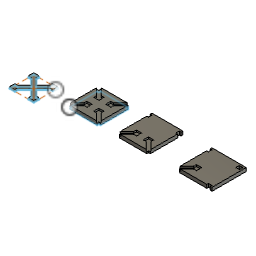
Maze_Alle_Module (Autodesk Fusion 360 design; units mm, degrees)
Autodesk Fusion 360 part; units mm, degrees
(part 1 of 2)
sketch "Skizze1" plane through (0, 0, 0) normal (0, 1, 0) x (1, 0, 0)
  line L0 (5, 0) -> (85, 0)
  line L1 (85, 0) -> (85, 5)
  line L2 (85, 5) -> (90, 5)
  line L3 (90, 5) -> (90, 85)
  line L4 (90, 85) -> (85, 85)
  line L5 (85, 85) -> (85, 90)
  line L6 (85, 90) -> (5, 90)
  line L7 (5, 90) -> (5, 85)
  line L8 (5, 85) -> (0, 85)
  line L9 (0, 85) -> (0, 5)
  line L10 (0, 5) -> (5, 5)
  line L11 (5, 5) -> (5, 0)
  line L12 (-35, 35) -> (35, 35) construction
  line L13 (35, 35) -> (35, -35) construction
  line L14 (35, -35) -> (-35, -35) construction
  line L15 (-35, -35) -> (-35, 35) construction
  line L16 (-35, 35) -> (35, -35) construction
  line L17 (35, 35) -> (-35, -35) construction
  line L18 (0, 0) -> (-3.5355, 3.5355) construction
  line L19 (-3.5355, 3.5355) -> (27.9289, 35) construction
  line L20 (-3.5355, 3.5355) -> (-35, -27.9289) construction
  line L21 (0, 0) -> (3.5355, -3.5355) construction
  line L22 (3.5355, -3.5355) -> (-27.9289, -35) construction
  line L23 (3.5355, -3.5355) -> (35.4271, 28.356) construction
  line L24 (0, 0) -> (3.5355, 3.5355) construction
  line L25 (3.5355, 3.5355) -> (35, -27.9289) construction
  line L26 (3.5355, 3.5355) -> (-27.9289, 35) construction
  line L27 (0, 0) -> (-3.5355, -3.5355) construction
  line L28 (-3.5355, -3.5355) -> (27.9289, -35) construction
  line L29 (-3.5355, -3.5355) -> (-35, 27.9289) construction
  line L30 (-35, 35) -> (-35, 20)
  line L31 (-35, 20) -> (-27.0711, 20)
  line L32 (-27.0711, 20) -> (-7.0711, 0)
  line L33 (-7.0711, 0) -> (-27.0709, -19.9998)
  line L34 (-27.0709, -19.9998) -> (-35, -19.9998)
  line L35 (-35, -19.9998) -> (-35, -35)
  line L36 (-35, -35) -> (-20, -35)
  line L37 (-20, -35) -> (-20, -27.0711)
  line L38 (-20, -27.0711) -> (0, -7.0711)
  line L39 (0, -7.0711) -> (19.9998, -27.0709)
  line L40 (19.9998, -35) -> (19.9998, -27.0709)
  line L41 (19.9998, -35) -> (35, -35)
  line L42 (35, -35) -> (35, -20)
  line L43 (27.0711, -20) -> (35, -20)
  line L44 (27.0711, -20) -> (7.0711, 0)
  line L45 (7.0711, 0) -> (27.0709, 19.9998)
  line L46 (35, 20) -> (35, 35)
  line L47 (35, 20) -> (27.0709, 19.9998)
  line L48 (35, 35) -> (20, 35)
  line L49 (20, 35) -> (20, 27.0711)
  line L50 (20, 27.0711) -> (0, 7.0711)
  line L51 (0, 7.0711) -> (-19.9998, 27.0709)
  line L52 (-20, 35) -> (-19.9998, 27.0709)
  line L53 (-20, 35) -> (-35, 35)
  line L54 (117.0711, -20) -> (97.0711, 0)
  line L55 (125, 35) -> (55, -35) construction
  line L56 (109.9998, -35) -> (125, -35)
  line L57 (125, 35) -> (110, 35)
  line L58 (90, 0) -> (93.5355, -3.5355) construction
  line L59 (93.5355, -3.5355) -> (125.4271, 28.356) construction
  line L60 (90, 7.0711) -> (70.0002, 27.0709)
  line L61 (90, 0) -> (86.4645, 3.5355) construction
  line L62 (125, 35) -> (125, -35) construction
  line L63 (117.0711, -20) -> (125, -20)
  line L64 (55, 35) -> (125, 35) construction
  line L65 (110, 35) -> (110, 27.0711)
  line L66 (125, 20) -> (125, 35)
  line L67 (109.9998, -35) -> (109.9998, -27.0709)
  line L68 (97.0711, 0) -> (117.0709, 19.9998)
  line L69 (125, -35) -> (125, -20)
  line L70 (90, 0) -> (93.5355, 3.5355) construction
  line L71 (93.5355, 3.5355) -> (125, -27.9289) construction
  line L72 (125, 20) -> (117.0709, 19.9998)
  line L73 (70, -27.0711) -> (90, -7.0711)
  line L74 (125, -35) -> (55, -35) construction
  line L75 (86.4645, 3.5355) -> (117.9289, 35) construction
  line L76 (93.5355, 3.5355) -> (62.0711, 35) construction
  line L77 (110, 27.0711) -> (90, 7.0711)
  line L78 (55, 35) -> (125, -35) construction
  line L79 (90, -7.0711) -> (109.9998, -27.0709)
  line L80 (93.5355, -3.5355) -> (62.0711, -35) construction
  line L81 (62.9289, 20) -> (82.9289, 0)
  line L82 (90, 0) -> (86.4645, -3.5355) construction
  line L83 (86.4645, -3.5355) -> (117.9289, -35) construction
  line L84 (86.4645, 3.5355) -> (55, -27.9289) construction
  line L85 (70, 35) -> (70.0002, 27.0709)
  line L86 (55, -35) -> (70, -35)
  line L87 (70, 35) -> (55, 35)
  line L88 (55, 20) -> (62.9289, 20)
  line L89 (55, -19.9998) -> (55, -35)
  line L90 (62.9291, -19.9998) -> (55, -19.9998)
  line L91 (55, 35) -> (55, 20)
  line L92 (86.4645, -3.5355) -> (55, 27.9289) construction
  line L93 (55, -35) -> (55, 35) construction
  line L94 (82.9289, 0) -> (62.9291, -19.9998)
  line L95 (70, -35) -> (70, -27.0711)
  line L96 (27.0711, 70) -> (7.0711, 90)
  line L97 (35, 125) -> (-35, 55) construction
  line L98 (19.9998, 55) -> (35, 55)
  line L99 (35, 125) -> (20, 125)
  line L100 (0, 90) -> (3.5355, 86.4645) construction
  line L101 (3.5355, 86.4645) -> (35.4271, 118.356) construction
  line L102 (0, 97.0711) -> (-19.9998, 117.0709)
  line L103 (0, 90) -> (-3.5355, 93.5355) construction
  line L104 (35, 125) -> (35, 55) construction
  line L105 (27.0711, 70) -> (35, 70)
  line L106 (-35, 125) -> (35, 125) construction
  line L107 (20, 125) -> (20, 117.0711)
  line L108 (35, 110) -> (35, 125)
  line L109 (19.9998, 55) -> (19.9998, 62.9291)
  line L110 (7.0711, 90) -> (27.0709, 109.9998)
  line L111 (35, 55) -> (35, 70)
  line L112 (0, 90) -> (3.5355, 93.5355) construction
  line L113 (3.5355, 93.5355) -> (35, 62.0711) construction
  line L114 (35, 110) -> (27.0709, 109.9998)
  line L115 (-20, 62.9289) -> (0, 82.9289)
  line L116 (35, 55) -> (-35, 55) construction
  line L117 (-3.5355, 93.5355) -> (27.9289, 125) construction
  line L118 (3.5355, 93.5355) -> (-27.9289, 125) construction
  line L119 (20, 117.0711) -> (0, 97.0711)
  line L120 (-35, 125) -> (35, 55) construction
  line L121 (0, 82.9289) -> (19.9998, 62.9291)
  line L122 (3.5355, 86.4645) -> (-27.9289, 55) construction
  line L123 (-27.0711, 110) -> (-7.0711, 90)
  line L124 (0, 90) -> (-3.5355, 86.4645) construction
  line L125 (-3.5355, 86.4645) -> (27.9289, 55) construction
  line L126 (-3.5355, 93.5355) -> (-35, 62.0711) construction
  line L127 (-20, 125) -> (-19.9998, 117.0709)
  line L128 (-35, 55) -> (-20, 55)
  line L129 (-20, 125) -> (-35, 125)
  line L130 (-35, 110) -> (-27.0711, 110)
  line L131 (-35, 70.0002) -> (-35, 55)
  line L132 (-27.0709, 70.0002) -> (-35, 70.0002)
  line L133 (-35, 125) -> (-35, 110)
  line L134 (-3.5355, 86.4645) -> (-35, 117.9289) construction
  line L135 (-35, 55) -> (-35, 125) construction
  line L136 (-7.0711, 90) -> (-27.0709, 70.0002)
  line L137 (-20, 55) -> (-20, 62.9289)
  line L138 (117.0711, 70) -> (97.0711, 90)
  line L139 (125, 125) -> (55, 55) construction
  line L140 (109.9998, 55) -> (125, 55)
  line L141 (125, 125) -> (110, 125)
  line L142 (90, 90) -> (93.5355, 86.4645) construction
  line L143 (93.5355, 86.4645) -> (125.4271, 118.356) construction
  line L144 (90, 97.0711) -> (70.0002, 117.0709)
  line L145 (90, 90) -> (86.4645, 93.5355) construction
  line L146 (125, 125) -> (125, 55) construction
  line L147 (117.0711, 70) -> (125, 70)
  line L148 (55, 125) -> (125, 125) construction
  line L149 (110, 125) -> (110, 117.0711)
  line L150 (125, 110) -> (125, 125)
  line L151 (109.9998, 55) -> (109.9998, 62.9291)
  line L152 (97.0711, 90) -> (117.0709, 109.9998)
  line L153 (125, 55) -> (125, 70)
  line L154 (90, 90) -> (93.5355, 93.5355) construction
  line L155 (93.5355, 93.5355) -> (125, 62.0711) construction
  line L156 (125, 110) -> (117.0709, 109.9998)
  line L157 (70, 62.9289) -> (90, 82.9289)
  line L158 (125, 55) -> (55, 55) construction
  line L159 (86.4645, 93.5355) -> (117.9289, 125) construction
  line L160 (93.5355, 93.5355) -> (62.0711, 125) construction
  line L161 (110, 117.0711) -> (90, 97.0711)
  line L162 (55, 125) -> (125, 55) construction
  line L163 (90, 82.9289) -> (109.9998, 62.9291)
  line L164 (93.5355, 86.4645) -> (62.0711, 55) construction
  line L165 (62.9289, 110) -> (82.9289, 90)
  line L166 (90, 90) -> (86.4645, 86.4645) construction
  line L167 (86.4645, 86.4645) -> (117.9289, 55) construction
  line L168 (86.4645, 93.5355) -> (55, 62.0711) construction
  line L169 (70, 125) -> (70.0002, 117.0709)
  line L170 (55, 55) -> (70, 55)
  line L171 (70, 125) -> (55, 125)
  line L172 (55, 110) -> (62.9289, 110)
  line L173 (55, 70.0002) -> (55, 55)
  line L174 (62.9291, 70.0002) -> (55, 70.0002)
  line L175 (55, 125) -> (55, 110)
  line L176 (86.4645, 86.4645) -> (55, 117.9289) construction
  line L177 (55, 55) -> (55, 125) construction
  line L178 (82.9289, 90) -> (62.9291, 70.0002)
  line L179 (70, 55) -> (70, 62.9289)
  line L180 (27.0711, -20) -> (7.0711, 0)
  line L181 (35, 35) -> (-35, -35) construction
  line L182 (19.9998, -35) -> (35, -35)
  line L183 (35, 35) -> (20, 35)
  line L184 (0, 0) -> (3.5355, -3.5355) construction
  line L185 (3.5355, -3.5355) -> (35.4271, 28.356) construction
  line L186 (0, 7.0711) -> (-19.9998, 27.0709)
  line L187 (0, 0) -> (-3.5355, 3.5355) construction
  line L188 (35, 35) -> (35, -35) construction
  line L189 (27.0711, -20) -> (35, -20)
  line L190 (-35, 35) -> (35, 35) construction
  line L191 (20, 35) -> (20, 27.0711)
  line L192 (35, 20) -> (35, 35)
  line L193 (19.9998, -35) -> (19.9998, -27.0709)
  line L194 (7.0711, 0) -> (27.0709, 19.9998)
  line L195 (35, -35) -> (35, -20)
  line L196 (0, 0) -> (3.5355, 3.5355) construction
  line L197 (3.5355, 3.5355) -> (35, -27.9289) construction
  line L198 (35, 20) -> (27.0709, 19.9998)
  line L199 (-20, -27.0711) -> (0, -7.0711)
  line L200 (35, -35) -> (-35, -35) construction
  line L201 (-3.5355, 3.5355) -> (27.9289, 35) construction
  line L202 (3.5355, 3.5355) -> (-27.9289, 35) construction
  line L203 (20, 27.0711) -> (0, 7.0711)
  line L204 (-35, 35) -> (35, -35) construction
  line L205 (0, -7.0711) -> (19.9998, -27.0709)
  line L206 (3.5355, -3.5355) -> (-27.9289, -35) construction
  line L207 (-27.0711, 20) -> (-7.0711, 0)
  line L208 (0, 0) -> (-3.5355, -3.5355) construction
  line L209 (-3.5355, -3.5355) -> (27.9289, -35) construction
  line L210 (-3.5355, 3.5355) -> (-35, -27.9289) construction
  line L211 (-20, 35) -> (-19.9998, 27.0709)
  line L212 (-35, -35) -> (-20, -35)
  line L213 (-20, 35) -> (-35, 35)
  line L214 (-35, 20) -> (-27.0711, 20)
  line L215 (-35, -19.9998) -> (-35, -35)
  line L216 (-27.0709, -19.9998) -> (-35, -19.9998)
  line L217 (-35, 35) -> (-35, 20)
  line L218 (-3.5355, -3.5355) -> (-35, 27.9289) construction
  line L219 (-35, -35) -> (-35, 35) construction
  line L220 (-7.0711, 0) -> (-27.0709, -19.9998)
  line L221 (-20, -35) -> (-20, -27.0711)
  line L222 (-20, 125) -> (-19.9998, 117.0709)
  line L223 (-27.0711, 110) -> (-7.0711, 90)
  line L224 (0, 90) -> (3.5355, 93.5355) construction
  line L225 (7.0711, 90) -> (27.0709, 109.9998)
  line L226 (20, 125) -> (20, 117.0711)
  line L227 (0, 97.0711) -> (-19.9998, 117.0709)
  line L228 (3.5355, 86.4645) -> (35.4271, 118.356) construction
  line L229 (-3.5355, 93.5355) -> (27.9289, 125) construction
  line L230 (35, 110) -> (27.0709, 109.9998)
  line L231 (0, 90) -> (-3.5355, 93.5355) construction
  line L232 (0, 90) -> (3.5355, 86.4645) construction
  line L233 (-3.5355, 86.4645) -> (-35, 117.9289) construction
  line L234 (0, 82.9289) -> (19.9998, 62.9291)
  line L235 (-3.5355, 86.4645) -> (27.9289, 55) construction
  line L236 (27.0711, 70) -> (7.0711, 90)
  line L237 (-35, 125) -> (35, 125) construction
  line L238 (3.5355, 86.4645) -> (-27.9289, 55) construction
  line L239 (35, 55) -> (35, 70)
  line L240 (-27.0709, 70.0002) -> (-35, 70.0002)
  line L241 (35, 55) -> (-35, 55) construction
  line L242 (5, 90) -> (5, 85)
  line L243 (35, 110) -> (35, 125)
  line L244 (0, 90) -> (-3.5355, 86.4645) construction
  line L245 (35, 125) -> (20, 125)
  line L246 (20, 117.0711) -> (0, 97.0711)
  line L247 (35, 125) -> (-35, 55) construction
  line L248 (5, 85) -> (0, 85)
  line L249 (27.0711, 70) -> (35, 70)
  line L250 (19.9998, 55) -> (19.9998, 62.9291)
  line L251 (-35, 125) -> (35, 55) construction
  line L252 (-35, 55) -> (-20, 55)
  line L253 (-35, 55) -> (-35, 125) construction
  line L254 (19.9998, 55) -> (35, 55)
  line L255 (-20, 55) -> (-20, 62.9289)
  line L256 (-35, 70.0002) -> (-35, 55)
  line L257 (-35, 125) -> (-35, 110)
  line L258 (-20, 125) -> (-35, 125)
  line L259 (-3.5355, 93.5355) -> (-35, 62.0711) construction
  line L260 (-35, 110) -> (-27.0711, 110)
  line L261 (3.5355, 93.5355) -> (35, 62.0711) construction
  line L262 (-7.0711, 90) -> (-27.0709, 70.0002)
  line L263 (3.5355, 93.5355) -> (-27.9289, 125) construction
  line L264 (35, 125) -> (35, 55) construction
  line L265 (-20, 62.9289) -> (0, 82.9289)
  dimension "d1" = 80
  dimension "d2" = 5
  dimension "d3" = 5
  dimension "d4" = 80
  dimension "d5" = 5
  dimension "d6" = 5
  dimension "d7" = 80
  dimension "d8" = 5
  dimension "d9" = 5
  dimension "d10" = 80
  dimension "d11" = 5
  dimension "d12" = 5
  dimension "d13" = 70
  dimension "d14" = 70
  dimension "d15" = 5
  dimension "d16" = 5
  dimension "d17" = 5
  dimension "d18" = 5
  dimension "d19" = 15
  dimension "d20" = 28.284
  dimension "d21" = 28.284
  dimension "d22" = 28.284
  dimension "d23" = 28.284
  dimension "d24" = 70
  dimension "d25" = 70
  dimension "d26" = 5
  dimension "d27" = 5
  dimension "d28" = 5
  dimension "d29" = 5
  dimension "d30" = 15
  dimension "d31" = 28.284
  dimension "d32" = 28.284
  dimension "d33" = 28.284
  dimension "d34" = 28.284
  dimension "d35" = 70
  dimension "d36" = 70
  dimension "d37" = 5
  dimension "d38" = 5
  dimension "d39" = 5
  dimension "d40" = 5
  dimension "d41" = 15
  dimension "d42" = 28.284
  dimension "d43" = 28.284
  dimension "d44" = 28.284
  dimension "d45" = 28.284
  dimension "d46" = 70
  dimension "d47" = 70
  dimension "d48" = 5
  dimension "d49" = 5
  dimension "d50" = 5
  dimension "d51" = 5
  dimension "d52" = 15
  dimension "d53" = 28.284
  dimension "d54" = 28.284
  dimension "d55" = 28.284
  dimension "d56" = 28.284
  dimension "d57" = 70
  dimension "d58" = 70
  dimension "d59" = 5
  dimension "d60" = 5
  dimension "d61" = 5
  dimension "d62" = 5
  dimension "d63" = 15
  dimension "d64" = 28.284
  dimension "d65" = 28.284
  dimension "d66" = 28.284
  dimension "d67" = 28.284
  dimension "d96" = 5
  dimension "d97" = 5
  dimension "d98" = 70
  dimension "d99" = 70
  dimension "d100" = 5
  dimension "d101" = 5
  dimension "d102" = 5
  dimension "d103" = 5
  dimension "d104" = 15
  dimension "d105" = 28.284
  dimension "d106" = 28.284
  dimension "d107" = 28.284
  dimension "d108" = 28.284
  constraint horizontal L0
  constraint perpendicular L0 L1
  constraint perpendicular L1 L2
  constraint perpendicular L0 L3
  constraint perpendicular L3 L4
  constraint perpendicular L0 L5
  constraint perpendicular L3 L6
  constraint perpendicular L6 L7
  constraint perpendicular L3 L8
  constraint perpendicular L6 L9
  constraint perpendicular L9 L10
  constraint perpendicular L0 L11
  constraint horizontal L12
  constraint vertical L13
  constraint horizontal L14
  constraint vertical L15
  constraint midpoint L17 L18.start
  constraint perpendicular L17 L18
  constraint coincident L12 L19.end
  constraint perpendicular L16 L19
  constraint coincident L15 L20.end
  constraint perpendicular L18 L20
  constraint perpendicular L17 L21
  constraint coincident L14 L22.end
  constraint perpendicular L21 L22
  constraint perpendicular L21 L23
  constraint coincident L17 L24.end
  constraint coincident L13 L25.end
  constraint perpendicular L24 L25
  constraint coincident L12 L26.end
  constraint perpendicular L24 L26
  constraint perpendicular L18 L27
  constraint coincident L14 L28.end
  constraint perpendicular L17 L28
  constraint coincident L15 L29.end
  constraint perpendicular L17 L29
  constraint perpendicular L12 L30
  constraint coincident L29 L31.end
  constraint perpendicular L15 L31
  constraint coincident L29 L32.end
  constraint coincident L20 L32.end
  constraint coincident L20 L33.end
  constraint coincident L15 L34.end
  constraint perpendicular L15 L34
  constraint coincident L14 L36.end
  constraint perpendicular L35 L36
  constraint coincident L22 L37.end
  constraint perpendicular L14 L37
  constraint coincident L28 L38.end
  constraint coincident L22 L38.end
  constraint perpendicular L28 L38
  constraint perpendicular L38 L39
  constraint coincident L14 L40.start
  constraint perpendicular L14 L40
  constraint coincident L13 L42.end
  constraint perpendicular L41 L42
  constraint coincident L25 L43.start
  constraint perpendicular L42 L43
  constraint coincident L25 L44.end
  constraint coincident L23 L44.end
  constraint perpendicular L23 L44
  constraint perpendicular L25 L45
  constraint coincident L13 L46.start
  constraint coincident L12 L48.end
  constraint perpendicular L13 L48
  constraint coincident L19 L49.end
  constraint perpendicular L12 L49
  constraint coincident L26 L50.end
  constraint coincident L19 L50.end
  constraint perpendicular L26 L50
  constraint perpendicular L50 L51
  constraint coincident L12 L52.start
  constraint horizontal L64
  constraint vertical L62
  constraint horizontal L74
  constraint vertical L93
  constraint midpoint L58.start L55
  constraint perpendicular L55 L61
  constraint coincident L75.end L64
  constraint perpendicular L75 L78
  constraint coincident L84.end L93
  constraint perpendicular L61 L84
  constraint perpendicular L55 L58
  constraint coincident L80.end L74
  constraint perpendicular L58 L80
  constraint perpendicular L58 L59
  constraint coincident L70.end L55
  constraint coincident L71.end L62
  constraint perpendicular L70 L71
  constraint coincident L76.end L64
  constraint perpendicular L70 L76
  constraint perpendicular L61 L82
  constraint coincident L83.end L74
  constraint perpendicular L55 L83
  constraint coincident L92.end L93
  constraint perpendicular L55 L92
  constraint perpendicular L64 L91
  constraint coincident L81.start L92
  constraint perpendicular L88 L93
  constraint coincident L81.end L92
  constraint coincident L81.end L84
  constraint coincident L90.start L84
  constraint coincident L89.start L93
  constraint perpendicular L90 L93
  constraint coincident L86.end L74
  constraint perpendicular L86 L89
  constraint coincident L73.start L80
  constraint perpendicular L74 L95
  constraint coincident L73.end L83
  constraint coincident L73.end L80
  constraint perpendicular L73 L83
  constraint perpendicular L73 L79
  constraint coincident L56.start L74
  constraint perpendicular L67 L74
  constraint coincident L63.end L62
  constraint perpendicular L56 L69
  constraint coincident L54.start L71
  constraint perpendicular L63 L69
  constraint coincident L54.end L71
  constraint coincident L54.end L59
  constraint perpendicular L54 L59
  constraint perpendicular L68 L71
  constraint coincident L66.start L62
  constraint coincident L57.end L64
  constraint perpendicular L57 L62
  constraint coincident L65.end L75
  constraint perpendicular L64 L65
  constraint coincident L60.start L76
  constraint coincident L60.start L75
  constraint perpendicular L76 L77
  constraint perpendicular L60 L77
  constraint coincident L85.start L64
  constraint horizontal L106
  constraint vertical L104
  constraint horizontal L116
  constraint vertical L135
  constraint midpoint L100.start L97
  constraint perpendicular L97 L103
  constraint coincident L117.end L106
  constraint perpendicular L117 L120
  constraint coincident L126.end L135
  constraint perpendicular L103 L126
  constraint perpendicular L97 L100
  constraint coincident L122.end L116
  constraint perpendicular L100 L122
  constraint perpendicular L100 L101
  constraint coincident L112.end L97
  constraint coincident L113.end L104
  constraint perpendicular L112 L113
  constraint coincident L118.end L106
  constraint perpendicular L112 L118
  constraint perpendicular L103 L124
  constraint coincident L125.end L116
  constraint perpendicular L97 L125
  constraint coincident L134.end L135
  constraint perpendicular L97 L134
  constraint perpendicular L106 L133
  constraint coincident L123.start L134
  constraint perpendicular L130 L135
  constraint coincident L123.end L134
  constraint coincident L123.end L126
  constraint coincident L132.start L126
  constraint coincident L131.start L135
  constraint perpendicular L132 L135
  constraint coincident L128.end L116
  constraint perpendicular L128 L131
  constraint coincident L115.start L122
  constraint perpendicular L116 L137
  constraint coincident L115.end L125
  constraint coincident L115.end L122
  constraint perpendicular L115 L125
  constraint perpendicular L115 L121
  constraint coincident L98.start L116
  constraint perpendicular L109 L116
  constraint coincident L105.end L104
  constraint perpendicular L98 L111
  constraint coincident L96.start L113
  constraint perpendicular L105 L111
  constraint coincident L96.end L113
  constraint coincident L96.end L101
  constraint perpendicular L96 L101
  constraint perpendicular L110 L113
  constraint coincident L108.start L104
  constraint coincident L99.end L106
  constraint perpendicular L99 L104
  constraint coincident L107.end L117
  constraint perpendicular L106 L107
  constraint coincident L102.start L118
  constraint coincident L102.start L117
  constraint perpendicular L118 L119
  constraint perpendicular L102 L119
  constraint coincident L127.start L106
  constraint horizontal L148
  constraint vertical L146
  constraint horizontal L158
  constraint vertical L177
  constraint midpoint L142.start L139
  constraint perpendicular L139 L145
  constraint coincident L159.end L148
  constraint perpendicular L159 L162
  constraint coincident L168.end L177
  constraint perpendicular L145 L168
  constraint perpendicular L139 L142
  constraint coincident L164.end L158
  constraint perpendicular L142 L164
  constraint perpendicular L142 L143
  constraint coincident L154.end L139
  constraint coincident L155.end L146
  constraint perpendicular L154 L155
  constraint coincident L160.end L148
  constraint perpendicular L154 L160
  constraint perpendicular L145 L166
  constraint coincident L167.end L158
  constraint perpendicular L139 L167
  constraint coincident L176.end L177
  constraint perpendicular L139 L176
  constraint perpendicular L148 L175
  constraint coincident L165.start L176
  constraint perpendicular L172 L177
  constraint coincident L165.end L176
  constraint coincident L165.end L168
  constraint coincident L174.start L168
  constraint coincident L173.start L177
  constraint perpendicular L174 L177
  constraint coincident L170.end L158
  constraint perpendicular L170 L173
  constraint coincident L157.start L164
  constraint perpendicular L158 L179
  constraint coincident L157.end L167
  constraint coincident L157.end L164
  constraint perpendicular L157 L167
  constraint perpendicular L157 L163
  constraint coincident L140.start L158
  constraint perpendicular L151 L158
  constraint coincident L147.end L146
  constraint perpendicular L140 L153
  constraint coincident L138.start L155
  constraint perpendicular L147 L153
  constraint coincident L138.end L155
  constraint coincident L138.end L143
  constraint perpendicular L138 L143
  constraint perpendicular L152 L155
  constraint coincident L150.start L146
  constraint coincident L141.end L148
  constraint perpendicular L141 L146
  constraint coincident L149.end L159
  constraint perpendicular L148 L149
  constraint coincident L144.start L160
  constraint coincident L144.start L159
  constraint perpendicular L160 L161
  constraint perpendicular L144 L161
  constraint coincident L169.start L148
  constraint horizontal L190
  constraint vertical L188
  constraint horizontal L200
  constraint vertical L219
  constraint midpoint L18.start L181
  constraint perpendicular L181 L187
  constraint coincident L19.end L190
  constraint perpendicular L201 L204
  constraint coincident L20.end L219
  constraint perpendicular L187 L210
  constraint perpendicular L181 L184
  constraint coincident L22.end L200
  constraint perpendicular L184 L206
  constraint perpendicular L184 L185
  constraint coincident L24.end L181
  constraint coincident L25.end L188
  constraint perpendicular L196 L197
  constraint coincident L26.end L190
  constraint perpendicular L196 L202
  constraint perpendicular L187 L208
  constraint coincident L28.end L200
  constraint perpendicular L181 L209
  constraint coincident L29.end L219
  constraint perpendicular L181 L218
  constraint perpendicular L190 L217
  constraint coincident L31.end L218
  constraint perpendicular L214 L219
  constraint coincident L32.end L218
  constraint coincident L32.end L210
  constraint coincident L33.end L210
  constraint coincident L34.end L219
  constraint perpendicular L216 L219
  constraint coincident L36.end L200
  constraint perpendicular L212 L215
  constraint coincident L37.end L206
  constraint perpendicular L200 L221
  constraint coincident L38.end L209
  constraint coincident L38.end L206
  constraint perpendicular L199 L209
  constraint perpendicular L199 L205
  constraint coincident L40.start L200
  constraint perpendicular L193 L200
  constraint coincident L42.end L188
  constraint perpendicular L182 L195
  constraint coincident L43.start L197
  constraint perpendicular L189 L195
  constraint coincident L44.end L197
  constraint coincident L44.end L185
  constraint perpendicular L180 L185
  constraint perpendicular L194 L197
  constraint coincident L46.start L188
  constraint coincident L48.end L190
  constraint perpendicular L183 L188
  constraint coincident L49.end L201
  constraint perpendicular L190 L191
  constraint coincident L50.end L202
  constraint coincident L50.end L201
  constraint perpendicular L202 L203
  constraint perpendicular L186 L203
  constraint coincident L52.start L190
  constraint horizontal L237
  constraint vertical L264
  constraint horizontal L241
  constraint vertical L253
  constraint midpoint L100.start L247
  constraint perpendicular L231 L247
  constraint coincident L117.end L237
  constraint perpendicular L229 L251
  constraint coincident L126.end L253
  constraint perpendicular L231 L259
  constraint perpendicular L232 L247
  constraint coincident L122.end L241
  constraint perpendicular L232 L238
  constraint perpendicular L228 L232
  constraint coincident L112.end L247
  constraint coincident L113.end L264
  constraint perpendicular L224 L261
  constraint coincident L118.end L237
  constraint perpendicular L224 L263
  constraint perpendicular L231 L244
  constraint coincident L125.end L241
  constraint perpendicular L235 L247
  constraint coincident L134.end L253
  constraint perpendicular L233 L247
  constraint perpendicular L237 L257
  constraint coincident L123.start L233
  constraint perpendicular L253 L260
  constraint coincident L123.end L233
  constraint coincident L123.end L259
  constraint coincident L132.start L259
  constraint coincident L131.start L253
  constraint perpendicular L240 L253
  constraint coincident L128.end L241
  constraint perpendicular L252 L256
  constraint coincident L115.start L238
  constraint perpendicular L241 L255
  constraint coincident L115.end L235
  constraint coincident L115.end L238
  constraint perpendicular L235 L265
  constraint perpendicular L234 L265
  constraint coincident L98.start L241
  constraint perpendicular L241 L250
  constraint coincident L105.end L264
  constraint perpendicular L239 L254
  constraint coincident L96.start L261
  constraint perpendicular L239 L249
  constraint coincident L96.end L261
  constraint coincident L96.end L228
  constraint perpendicular L228 L236
  constraint perpendicular L225 L261
  constraint coincident L108.start L264
  constraint coincident L99.end L237
  constraint perpendicular L245 L264
  constraint coincident L107.end L229
  constraint perpendicular L226 L237
  constraint coincident L102.start L263
  constraint coincident L102.start L229
  constraint perpendicular L246 L263
  constraint perpendicular L227 L246
  constraint coincident L127.start L237
  measures "d1" distance of L0.start L0.end
  measures "d2" distance of L0.end L1.end
  measures "d3" distance of L1.end L2.end
  measures "d4" distance of L2.end L3.end
  measures "d5" distance of L3.end L4.end
  measures "d6" distance of L4.end L5.end
  measures "d7" distance of L5.end L6.end
  measures "d8" distance of L6.end L7.end
  measures "d9" distance of L7.end L8.end
  measures "d10" distance of L8.end L9.end
  measures "d11" distance of L9.end L10.end
  measures "d12" distance of L10.end L0.start
  measures "d13" distance of L12.start L12.end
  measures "d14" distance of L12.start L14.end
  measures "d15" distance of L18.start L18.end
  measures "d16" distance of L18.start L21.end
  measures "d17" distance of L18.start L24.end
  measures "d18" distance of L18.start L27.end
  measures "d19" distance of L12.start L30.end
  measures "d20" distance of L32.end L33.end
  measures "d21" distance of L38.end L39.end
  measures "d22" distance of L44.end L45.end
  measures "d23" distance of L50.end L51.end
  measures "d24" distance of L64.start L55.start
  measures "d25" distance of L64.start L55.end
  measures "d26" distance of L58.start L61.end
  measures "d27" distance of L58.start L58.end
  measures "d28" distance of L58.start L70.end
  measures "d29" distance of L58.start L82.end
  measures "d30" distance of L64.start L88.start
  measures "d31" distance of L90.start L81.end
  measures "d32" distance of L73.end L67.end
  measures "d33" distance of L68.end L54.end
  measures "d34" distance of L60.start L60.end
  measures "d35" distance of L106.start L97.start
  measures "d36" distance of L106.start L97.end
  measures "d37" distance of L100.start L103.end
  measures "d38" distance of L100.start L100.end
  measures "d39" distance of L100.start L112.end
  measures "d40" distance of L100.start L124.end
  measures "d41" distance of L106.start L130.start
  measures "d42" distance of L132.start L123.end
  measures "d43" distance of L115.end L109.end
  measures "d44" distance of L110.end L96.end
  measures "d45" distance of L102.start L102.end
  measures "d46" distance of L148.start L139.start
  measures "d47" distance of L148.start L139.end
  measures "d48" distance of L142.start L145.end
  measures "d49" distance of L142.start L142.end
  measures "d50" distance of L142.start L154.end
  measures "d51" distance of L142.start L166.end
  measures "d52" distance of L148.start L172.start
  measures "d53" distance of L174.start L165.end
  measures "d54" distance of L157.end L151.end
  measures "d55" distance of L152.end L138.end
  measures "d56" distance of L144.start L144.end
  measures "d57" distance of L12.start L12.end
  measures "d58" distance of L12.start L14.end
  measures "d59" distance of L18.start L18.end
  measures "d60" distance of L18.start L21.end
  measures "d61" distance of L18.start L24.end
  measures "d62" distance of L18.start L27.end
  measures "d63" distance of L12.start L30.end
  measures "d64" distance of L33.end L32.end
  measures "d65" distance of L38.end L39.end
  measures "d66" distance of L45.end L44.end
  measures "d67" distance of L50.end L51.end
  measures "d96" distance of L7.end L6.end
  measures "d97" distance of L8.end L7.end
  measures "d98" distance of L97.start L106.start
  measures "d99" distance of L97.end L106.start
  measures "d100" distance of L100.start L103.end
  measures "d101" distance of L100.start L100.end
  measures "d102" distance of L112.end L100.start
  measures "d103" distance of L100.start L124.end
  measures "d104" distance of L106.start L130.start
  measures "d105" distance of L132.start L123.end
  measures "d106" distance of L115.end L109.end
  measures "d107" distance of L96.end L110.end
  measures "d108" distance of L102.end L102.start
extrude "Extrusion1" add sketch "Skizze1" along normal blind 10 contours L0 L3 L6 L9 L45 L46 L47 L48 L49 L50 L60 L81 L85 L87 L88 L91 L96 L98 L105 L109 L111 L121 L157 L170 L173 L174 L178 L179 L183 L191 L192 L194 L198 L203 L234 L236 L239 L249 L250 L254 makes body 1
sketch "Skizze2" plane through (0, 0, 0) normal (0, 1, 0) x (1, 0, 0)
  line L0 (0, 5) -> (5, 5)
  line L1 (5, 5) -> (5, 0)
  line L2 (5, 0) -> (85, 0)
  line L3 (85, 0) -> (85, 5)
  line L4 (85, 5) -> (90, 5)
  line L5 (90, 5) -> (90, 85)
  line L6 (90, 85) -> (85, 85)
  line L7 (85, 85) -> (85, 90)
  line L8 (85, 90) -> (5, 90)
  line L9 (5, 90) -> (5, 85)
  line L10 (5, 85) -> (0, 85)
  line L11 (0, 85) -> (0, 5)
  dimension "d70" = 80
  dimension "d71" = 5
  dimension "d72" = 5
  dimension "d73" = 80
  dimension "d74" = 5
  dimension "d75" = 5
  dimension "d76" = 80
  dimension "d77" = 5
  dimension "d78" = 5
  dimension "d79" = 80
  constraint horizontal L0
  constraint perpendicular L0 L1
  constraint perpendicular L1 L2
  constraint perpendicular L2 L3
  constraint perpendicular L1 L4
  constraint perpendicular L2 L5
  constraint perpendicular L5 L6
  constraint perpendicular L2 L7
  constraint perpendicular L5 L8
  constraint perpendicular L8 L9
  constraint perpendicular L5 L10
  constraint perpendicular L8 L11
  measures "d70" distance of L1.end L2.end
  measures "d71" distance of L2.end L3.end
  measures "d72" distance of L3.end L4.end
  measures "d73" distance of L4.end L5.end
  measures "d74" distance of L5.end L6.end
  measures "d75" distance of L6.end L7.end
  measures "d76" distance of L7.end L8.end
  measures "d77" distance of L8.end L9.end
  measures "d78" distance of L9.end L10.end
  measures "d79" distance of L10.end L0.start
extrude "Extrusion2" add sketch "Skizze2" along normal blind 5 bodies 1
sketch "Skizze3" plane through (0, 0, 0) normal (0, 1, 0) x (1, 0, 0)
  line L0 (-72.9289, -20) -> (-92.9289, 0)
  line L1 (-65, 35) -> (-135, -35) construction
  line L2 (-80.0002, -35) -> (-65, -35)
  line L3 (-65, 35) -> (-80, 35)
  line L4 (-100, 0) -> (-96.4645, -3.5355) construction
  line L5 (-96.4645, -3.5355) -> (-64.5729, 28.356) construction
  line L6 (-100, 7.0711) -> (-119.9998, 27.0709)
  line L7 (-100, 0) -> (-103.5355, 3.5355) construction
  line L8 (-65, 35) -> (-65, -35) construction
  line L9 (-72.9289, -20) -> (-65, -20)
  line L10 (-135, 35) -> (-65, 35) construction
  line L11 (-80, 35) -> (-80, 27.0711)
  line L12 (-65, 20) -> (-65, 35)
  line L13 (-80.0002, -35) -> (-80.0002, -27.0709)
  line L14 (-92.9289, 0) -> (-72.9291, 19.9998)
  line L15 (-65, -35) -> (-65, -20)
  line L16 (-100, 0) -> (-96.4645, 3.5355) construction
  line L17 (-96.4645, 3.5355) -> (-65, -27.9289) construction
  line L18 (-65, 20) -> (-72.9291, 19.9998)
  line L19 (-120, -27.0711) -> (-100, -7.0711)
  line L20 (-65, -35) -> (-135, -35) construction
  line L21 (-103.5355, 3.5355) -> (-72.0711, 35) construction
  line L22 (-96.4645, 3.5355) -> (-127.9289, 35) construction
  line L23 (-80, 27.0711) -> (-100, 7.0711)
  line L24 (-135, 35) -> (-65, -35) construction
  line L25 (-100, -7.0711) -> (-80.0002, -27.0709)
  line L26 (-96.4645, -3.5355) -> (-127.9289, -35) construction
  line L27 (-127.0711, 20) -> (-107.0711, 0)
  line L28 (-100, 0) -> (-103.5355, -3.5355) construction
  line L29 (-103.5355, -3.5355) -> (-72.0711, -35) construction
  line L30 (-103.5355, 3.5355) -> (-135, -27.9289) construction
  line L31 (-120, 35) -> (-119.9998, 27.0709)
  line L32 (-135, -35) -> (-120, -35)
  line L33 (-120, 35) -> (-135, 35)
  line L34 (-135, 20) -> (-127.0711, 20)
  line L35 (-135, -19.9998) -> (-135, -35)
  line L36 (-127.0709, -19.9998) -> (-135, -19.9998)
  line L37 (-135, 35) -> (-135, 20)
  line L38 (-103.5355, -3.5355) -> (-135, 27.9289) construction
  line L39 (-135, -35) -> (-135, 35) construction
  line L40 (-107.0711, 0) -> (-127.0709, -19.9998)
  line L41 (-120, -35) -> (-120, -27.0711)
  line L42 (-120.1, 34.9) -> (-120.0998, 27.0295)
  line L43 (-100, 6.9296) -> (-120.0998, 27.0295)
  line L44 (-79.9, 27.0296) -> (-100, 6.9296)
  line L45 (-79.9, 34.9) -> (-79.9, 27.0296)
  line L46 (-65.1, 34.9) -> (-79.9, 34.9)
  line L47 (-65.1, 20.1) -> (-65.1, 34.9)
  line L48 (-65.1, 20.1) -> (-72.9705, 20.0998)
  line L49 (-93.0704, 0) -> (-72.9705, 20.0998)
  line L50 (-72.9704, -20.1) -> (-93.0704, 0)
  line L51 (-72.9704, -20.1) -> (-65.1, -20.1)
  line L52 (-65.1, -34.9) -> (-65.1, -20.1)
  line L53 (-79.9002, -34.9) -> (-65.1, -34.9)
  line L54 (-79.9002, -34.9) -> (-79.9002, -27.0295)
  line L55 (-100, -6.9296) -> (-79.9002, -27.0295)
  line L56 (-120.1, -27.0296) -> (-100, -6.9296)
  line L57 (-120.1, -34.9) -> (-120.1, -27.0296)
  line L58 (-134.9, -34.9) -> (-120.1, -34.9)
  line L59 (-134.9, -20.0998) -> (-134.9, -34.9)
  line L60 (-127.0295, -20.0998) -> (-134.9, -20.0998)
  line L61 (-106.9296, 0) -> (-127.0295, -20.0998)
  line L62 (-127.0296, 20.1) -> (-106.9296, 0)
  line L63 (-134.9, 20.1) -> (-127.0296, 20.1)
  line L64 (-134.9, 34.9) -> (-134.9, 20.1)
  line L65 (-120.1, 34.9) -> (-134.9, 34.9)
  dimension "d82" = 70
  dimension "d83" = 70
  dimension "d84" = 5
  dimension "d85" = 5
  dimension "d86" = 5
  dimension "d87" = 5
  dimension "d88" = 15
  dimension "d89" = 28.284
  dimension "d90" = 28.284
  dimension "d91" = 28.284
  dimension "d92" = 28.284
  dimension "d93" = -0.1
  constraint horizontal L10
  constraint vertical L8
  constraint horizontal L20
  constraint vertical L39
  constraint midpoint L4.start L1
  constraint perpendicular L1 L7
  constraint coincident L21.end L10
  constraint perpendicular L21 L24
  constraint coincident L30.end L39
  constraint perpendicular L7 L30
  constraint perpendicular L1 L4
  constraint coincident L26.end L20
  constraint perpendicular L4 L26
  constraint perpendicular L4 L5
  constraint coincident L16.end L1
  constraint coincident L17.end L8
  constraint perpendicular L16 L17
  constraint coincident L22.end L10
  constraint perpendicular L16 L22
  constraint perpendicular L7 L28
  constraint coincident L29.end L20
  constraint perpendicular L1 L29
  constraint coincident L38.end L39
  constraint perpendicular L1 L38
  constraint perpendicular L10 L37
  constraint coincident L27.start L38
  constraint perpendicular L34 L39
  constraint coincident L27.end L38
  constraint coincident L27.end L30
  constraint coincident L36.start L30
  constraint coincident L35.start L39
  constraint perpendicular L36 L39
  constraint coincident L32.end L20
  constraint perpendicular L32 L35
  constraint coincident L19.start L26
  constraint perpendicular L20 L41
  constraint coincident L19.end L29
  constraint coincident L19.end L26
  constraint perpendicular L19 L29
  constraint perpendicular L19 L25
  constraint coincident L2.start L20
  constraint perpendicular L13 L20
  constraint coincident L9.end L8
  constraint perpendicular L2 L15
  constraint coincident L0.start L17
  constraint perpendicular L9 L15
  constraint coincident L0.end L17
  constraint coincident L0.end L5
  constraint perpendicular L0 L5
  constraint perpendicular L14 L17
  constraint coincident L12.start L8
  constraint coincident L3.end L10
  constraint perpendicular L3 L8
  constraint coincident L11.end L21
  constraint perpendicular L10 L11
  constraint coincident L6.start L22
  constraint coincident L6.start L21
  constraint perpendicular L22 L23
  constraint perpendicular L6 L23
  constraint coincident L31.start L10
  measures "d82" distance of L10.start L1.start
  measures "d83" distance of L10.start L1.end
  measures "d84" distance of L4.start L7.end
  measures "d85" distance of L4.start L4.end
  measures "d86" distance of L4.start L16.end
  measures "d87" distance of L4.start L28.end
  measures "d88" distance of L10.start L34.start
  measures "d89" distance of L36.start L27.end
  measures "d90" distance of L19.end L13.end
  measures "d91" distance of L14.end L0.end
  measures "d92" distance of L6.start L6.end
extrude "Extrusion3" add sketch "Skizze3" along normal blind 4.8 separate body contours L42 L43 L44 L45 L46 L47 L48 L49 L50 L51 L52 L53 L54 L55 L56 L57 L58 L59 L60 L61 L62 L63 L64 L65 makes body 2
copy_body "Körper kopieren/einfügen1" bodies 1 makes body 3